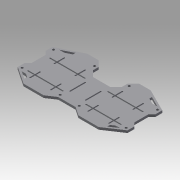
# Autodesk Inventor part: Board_Support
Saved by Autodesk Inventor 2016 (Build 200138000, 138)
## iProperties
Created: 2015-09-29
Part Number: Board_Support
Material: Générique
Document SubType Name: Modeling
Designer: Logan
Density: 1 g/cm^3
Appearance: Par défaut
Author: Logan
Autodesk Inventor part; units mm, degrees
ref_plane "YZ Plane" through (0, 0, 0) normal (1, 0, 0) x (0, 1, 0)
ref_plane "XZ Plane" through (0, 0, 0) normal (0, 1, 0) x (-1, 0, 0)
ref_plane "XY Plane" through (0, 0, 0) normal (0, 0, 1) x (1, 0, 0)
sketch "Esquisse1" plane through (0, 0, 0) normal (0, 0, 1) x (1, 0, 0)
  line L0 (-190, -60) -> (-190, 60)
  line L1 (190, 60) -> (190, -60)
  line L2 (-110, 100) -> (-190, 60)
  line L3 (110, 100) -> (190, 60)
  line L4 (-190, -60) -> (-130, -100)
  line L5 (130, -100) -> (190, -60)
  line L6 (70, 100) -> (110, 100)
  line L7 (130, -100) -> (60, -100)
  line L8 (-60, -100) -> (-130, -100)
  line L9 (30, 40) -> (-30, 40)
  line L10 (-110, 100) -> (-70, 100)
  line L11 (60, 100) -> (110, 100)
  line L12 (-60, -100) -> (-30, -80)
  line L13 (-30, -80) -> (30, -80)
  line L14 (30, -80) -> (60, -100)
  line L15 (-50, 60) -> (-50, 80)
  line L16 (50, 60) -> (50, 80)
  line L17 (-30, 40) -> (-50, 60)
  line L18 (30, 40) -> (50, 60)
  line L19 (-70, 100) -> (-50, 80)
  line L20 (70, 100) -> (50, 80)
  point P0 (0, 0)
  point P1 (-60, 100)
  point P2 (-50, 40)
  point P3 (50, 40)
  point P4 (-50, 100)
  point P5 (50, 100)
  dimension "d204" = 60
  dimension "d207" = 50
  dimension "d208" = 50
  dimension "d211" = 20
  dimension "d212" = 30
  dimension "d213" = 30
  dimension "d214" = 20
  dimension "d215" = 20
  dimension "d216" = 20
  dimension "d217" = 20
  dimension "d218" = 20
  dimension "d219" = 20
  dimension "d220" = 20
  dimension "d221" = 20
  dimension "d227" = 80
  dimension "d228" = 40
  dimension "d229" = 60
  dimension "d230" = 40
  dimension "d231" = 80
  dimension "d232" = 40
  dimension "d233" = 60
  dimension "d234" = 380
  dimension "d235" = 190
  dimension "d236" = 30
  dimension "d250" = 60
  dimension "d251" = 40
  constraints: 42 end point, 10 point on line, 7 parallel, 3 horizontal, 2 collinear, 2 perpendicular, 2 vertical
  measures "d204" distance between parallel lines of L9 L10
  measures "d207" horizontal distance of point (0, 0) point (50, 40)
  measures "d208" horizontal distance of point (0, 0) point (-50, 40)
  measures "d211" distance between parallel lines of L8 L13
  measures "d212" horizontal distance of L12.end L8.start
  measures "d213" horizontal distance of L7.end L13.end
  measures "d214" distance of L9.end point (-50, 40)
  measures "d215" distance of L15.start point (-50, 40)
  measures "d216" distance of L9.start point (50, 40)
  measures "d217" distance of L16.start point (50, 40)
  measures "d218" distance of L10.end point (-50, 100)
  measures "d219" distance of L15.end point (-50, 100)
  measures "d220" distance of L6.start point (50, 100)
  measures "d221" distance of L16.end point (50, 100)
  measures "d227" horizontal distance of L2.start L0.end
  measures "d228" vertical distance of L2.start L0.end
  measures "d229" horizontal distance of L0.start L4.end
  measures "d230" vertical distance of L0.start L4.end
  measures "d231" horizontal distance of L3.start L1.start
  measures "d232" vertical distance of L3.start L1.start
  measures "d233" distance of L12.end L13.end
  measures "d234" distance between parallel lines of L1 L0
  measures "d235" distance from line of point (0, 0) L0
  measures "d236" horizontal distance of point (0, 0) L13.end
  measures "d250" horizontal distance of L5.start L1.end
  measures "d251" vertical distance of L5.start L1.end
extrude "Plaque" add sketch "Esquisse1" along normal blind 8
sketch "Esquisse8" plane through (0, 0, 8) normal (0, 0, 1) x (1, 0, 0)
  line L0 (-178, -30) -> (-190, -30)
  line L1 (-190, -30) -> (-190, 30)
  line L2 (-190, 30) -> (-178, 30)
  line L3 (-178, 30) -> (-178, -30)
  line L4 (-178, -30) -> (-190, 30) construction
  line L5 (-190, -30) -> (-178, 30) construction
  line L6 (0, 43.7993) -> (0, -83.0015)
  line L7 (178, -30) -> (190, -30)
  line L8 (190, -30) -> (190, 30)
  line L9 (190, 30) -> (178, 30)
  line L10 (178, 30) -> (178, -30)
  line L11 (178, -30) -> (190, 30) construction
  line L12 (190, -30) -> (178, 30) construction
  point P0 (0, 0)
  point P1 (-184, 0)
  point P2 (184, 0)
  dimension "d106" = 60
  dimension "d107" = 12
  dimension "d108" = 178
  dimension "d191" = 30
  constraints: 26 end point, 5 symmetric about line, 4 midpoint, 2 parallel, 1 horizontal, 1 perpendicular, 1 vertical
  measures "d106" distance of L2.end L0.start
  measures "d107" distance of L1.end L2.end
  measures "d108" distance from line of point (0, 0) L3
  measures "d191" distance from line of point (0, 0) L2
extrude "Passage_Encodeur" cut sketch "Esquisse8" against normal up to surface (8 mm away)
chamfer "Passage_cable" distance 6 angle 45 8 edges at (-178, 30, 4) (-178, -30, 4) (178, 30, 4) (178, -30, 4) (190, 30, 4) (-190, 30, 4) (-190, -30, 4) (190, -30, 4)
sketch "Esquisse12" plane through (0, 0, 8) normal (0, 0, 1) x (1, 0, 0)
  line L0 (178, -24) -> (190, -36) projected
  line L1 (178, -24) -> (178, 24) projected
  line L2 (190, 36) -> (178, 24) projected
  line L3 (190, 36) -> (190, 60) projected
  line L4 (190, 60) -> (110, 100) projected
  line L5 (110, 100) -> (70, 100) projected
  line L6 (70, 100) -> (50, 80) projected
  line L7 (50, 80) -> (50, 60) projected
  line L8 (50, 60) -> (30, 40) projected
  line L9 (30, 40) -> (-30, 40) projected
  line L10 (-30, 40) -> (-50, 60) projected
  line L11 (-50, 60) -> (-50, 80) projected
  line L12 (-50, 80) -> (-70, 100) projected
  line L13 (-70, 100) -> (-110, 100) projected
  line L14 (-110, 100) -> (-190, 60) projected
  line L15 (-190, 60) -> (-190, 36) projected
  line L16 (-178, 24) -> (-190, 36) projected
  line L17 (-178, 24) -> (-178, -24) projected
  line L18 (-190, -36) -> (-178, -24) projected
  line L19 (-190, -36) -> (-190, -60) projected
  line L20 (-190, -60) -> (-130, -100) projected
  line L21 (-130, -100) -> (-60, -100) projected
  line L22 (-60, -100) -> (-30, -80) projected
  line L23 (-30, -80) -> (30, -80) projected
  line L24 (30, -80) -> (60, -100) projected
  line L25 (60, -100) -> (130, -100) projected
  line L26 (130, -100) -> (190, -60) projected
  line L27 (190, -60) -> (190, -36) projected
  line L28 (-180, 53.8197) -> (-107.6393, 90)
  line L29 (-107.6393, 90) -> (-74.1421, 90)
  line L30 (-74.1421, 90) -> (-60, 75.8579)
  line L31 (-60, 75.8579) -> (-60, 55.8579)
  line L32 (-60, 55.8579) -> (-34.1421, 30)
  line L33 (-34.1421, 30) -> (34.1421, 30)
  line L34 (34.1421, 30) -> (60, 55.8579)
  line L35 (60, 55.8579) -> (60, 75.8579)
  line L36 (60, 75.8579) -> (74.1421, 90)
  line L37 (74.1421, 90) -> (107.6393, 90)
  line L38 (107.6393, 90) -> (180, 53.8197)
  line L39 (180, 53.8197) -> (180, 40.1421)
  line L40 (180, 40.1421) -> (168, 28.1421)
  line L41 (168, 28.1421) -> (168, -28.1421)
  line L42 (168, -28.1421) -> (180, -40.1421)
  line L43 (180, -40.1421) -> (180, -54.6482)
  line L44 (180, -54.6482) -> (126.9722, -90)
  line L45 (126.9722, -90) -> (63.0278, -90)
  line L46 (63.0278, -90) -> (33.0278, -70)
  line L47 (33.0278, -70) -> (-33.0278, -70)
  line L48 (-33.0278, -70) -> (-63.0278, -90)
  line L49 (-63.0278, -90) -> (-126.9722, -90)
  line L50 (-126.9722, -90) -> (-180, -54.6482)
  line L51 (-180, -54.6482) -> (-180, -40.1421)
  line L52 (-180, -40.1421) -> (-168, -28.1421)
  line L53 (-168, -28.1421) -> (-168, 28.1421)
  line L54 (-168, 28.1421) -> (-180, 40.1421)
  line L55 (-180, 40.1421) -> (-180, 53.8197)
  point P0 (0, 0)
  dimension "d263" = 10
  constraints: 56 end point, 27 other
  measures "d263" distance between parallel lines of L14 L28
hole "Support_Etage" at (-180, 53.8197, 8) at (180, 53.8197, 8) at (180, -54.6482, 8) at (-180, -54.6482, 8) at (-60, 75.8579, 8) at (60, 75.8579, 8) at (33.0278, -70, 8) at (-33.0278, -70, 8) direction (0, 0, -1) diameter 8 end through all
sketch "Esquisse16" plane through (0, 0, 8) normal (0, 0, 1) x (1, 0, 0)
  line L0 (-110, 100) -> (-190, 60) projected
  line L1 (-169.9266, 63.3285) -> (-132.3607, 82.1115)
  line L2 (-132.3607, 82.1115) -> (-132.3607, 82.1115)
  line L3 (-132.3607, 73.1672) -> (-152.0381, 63.3285)
  line L4 (-169.9266, 63.3285) -> (-169.9266, 63.3285)
  line L5 (-132.3607, 82.1115) -> (-132.3607, 73.1672)
  line L6 (-152.0381, 63.3285) -> (-169.9266, 63.3285)
  line L7 (-50, 60) -> (-50, 80) projected
  line L8 (-70, 100) -> (-110, 100) projected
  line L9 (-190, -60) -> (-130, -100) projected
  line L10 (-169.9266, -66.1711) -> (-143.301, -83.9216)
  line L11 (-143.301, -83.9216) -> (-143.301, -83.9216)
  line L12 (-143.301, -74.3068) -> (-155.5044, -66.1711)
  line L13 (-169.9266, -66.1711) -> (-169.9266, -66.1711)
  line L14 (-155.5044, -66.1711) -> (-169.9266, -66.1711)
  line L15 (-143.301, -83.9216) -> (-143.301, -74.3068)
  line L16 (-190, -36) -> (-190, -60) projected
  line L17 (-130, -100) -> (-60, -100) projected
  line L18 (0, 0) -> (0, -41.1993)
  line L19 (110, 100) -> (190, 60)
  line L20 (169.9266, 63.3285) -> (132.3607, 82.1115)
  line L21 (132.3607, 82.1115) -> (132.3607, 82.1115)
  line L22 (132.3607, 73.1672) -> (152.0381, 63.3285)
  line L23 (169.9266, 63.3285) -> (169.9266, 63.3285)
  line L24 (132.3607, 82.1115) -> (132.3607, 73.1672)
  line L25 (152.0381, 63.3285) -> (169.9266, 63.3285)
  line L26 (50, 60) -> (50, 80)
  line L27 (70, 100) -> (110, 100)
  line L28 (190, -60) -> (130, -100)
  line L29 (169.9266, -66.1711) -> (143.301, -83.9216)
  line L30 (143.301, -83.9216) -> (143.301, -83.9216)
  line L31 (143.301, -74.3068) -> (155.5044, -66.1711)
  line L32 (169.9266, -66.1711) -> (169.9266, -66.1711)
  line L33 (155.5044, -66.1711) -> (169.9266, -66.1711)
  line L34 (143.301, -83.9216) -> (143.301, -74.3068)
  line L35 (190, -36) -> (190, -60)
  line L36 (130, -100) -> (60, -100)
  point P0 (-128.783, 74.956)
  point P1 (-166.3489, 56.1731)
  point P2 (-138.8634, -77.2652)
  point P3 (-165.489, -59.5147)
  point P4 (128.783, 74.956)
  point P5 (166.3489, 56.1731)
  point P6 (138.8634, -77.2652)
  point P7 (165.489, -59.5147)
  dimension "d310" = 8
  dimension "d311" = 6
  dimension "d312" = 42
  dimension "d313" = 28
  dimension "d316" = 8
  dimension "d319" = 8
  dimension "d320" = 8
  dimension "d323" = 32
  dimension "d324" = 6
  dimension "d326" = 8
  dimension "d327" = 8
  dimension "d329" = 0
  constraints: 62 end point, 25 symmetric about line, 16 point on line, 10 parallel, 2 perpendicular, 1 vertical
  measures "d310" distance between parallel lines of L1 L3
  measures "d311" distance between parallel lines of L0 L1
  measures "d312" distance between parallel lines of L2 L4
  measures "d313" distance from line of L0.start L2
  measures "d316" distance of L2.end point (-128.783, 74.956)
  measures "d319" distance of L4.start point (-166.349, 56.173)
  measures "d320" distance between parallel lines of L12 L10
  measures "d323" distance between parallel lines of L11 L13
  measures "d324" distance between parallel lines of L9 L10
  measures "d326" distance of L13.start point (-165.489, -59.515)
  measures "d327" distance of L11.end point (-138.863, -77.265)
  measures "d329" horizontal distance of L1.start L10.start
extrude "Extrusion6" cut sketch "Esquisse16" against normal up to next
sketch "Esquisse17" plane through (0, 0, 8) normal (0, 0, 1) x (1, 0, 0)
  line L0 (160.48, 22.48) -> (160.48, -53.72)
  line L1 (-30, -80) -> (30, -80) projected
  line L2 (30, 40) -> (-30, 40) projected
  line L3 (178, -24) -> (178, 24) projected
  line L4 (-178, 24) -> (-178, -24) projected
  line L5 (-160.48, 22.48) -> (-40.48, 22.48) construction
  line L6 (-160.48, 20.48) -> (-40.48, 20.48)
  line L7 (-40.48, 24.48) -> (-160.48, 24.48)
  arc A0 (-160.48, 24.48) -> (-160.48, 20.48) centre (-160.48, 22.48) ccw
  arc A1 (-40.48, 20.48) -> (-40.48, 24.48) centre (-40.48, 22.48) ccw
  line L8 (-160.48, -53.72) -> (-40.48, -53.72) construction
  line L9 (-160.48, -55.72) -> (-40.48, -55.72)
  line L10 (-40.48, -51.72) -> (-160.48, -51.72)
  arc A2 (-160.48, -51.72) -> (-160.48, -55.72) centre (-160.48, -53.72) ccw
  arc A3 (-40.48, -55.72) -> (-40.48, -51.72) centre (-40.48, -53.72) ccw
  line L11 (0, 0) -> (0, -19.5991)
  line L12 (-40.48, 24.48) -> (-40.48, 20.48)
  line L13 (-40.48, -51.72) -> (-40.48, -55.72)
  line L14 (-160.48, -53.72) -> (-160.48, -51.72)
  line L15 (-160.48, 20.48) -> (-160.48, 22.48)
  line L16 (-160.48, 22.48) -> (-40.48, 22.48)
  line L17 (-40.48, -53.72) -> (-160.48, -53.72)
  line L18 (160.48, 22.48) -> (40.48, 22.48) construction
  line L19 (160.48, 20.48) -> (40.48, 20.48)
  line L20 (40.48, 24.48) -> (160.48, 24.48)
  arc A4 (160.48, 20.48) -> (160.48, 24.48) centre (160.48, 22.48) ccw
  arc A5 (40.48, 24.48) -> (40.48, 20.48) centre (40.48, 22.48) ccw
  line L21 (160.48, -53.72) -> (40.48, -53.72) construction
  line L22 (160.48, -55.72) -> (40.48, -55.72)
  line L23 (40.48, -51.72) -> (160.48, -51.72)
  arc A6 (160.48, -55.72) -> (160.48, -51.72) centre (160.48, -53.72) ccw
  arc A7 (40.48, -51.72) -> (40.48, -55.72) centre (40.48, -53.72) ccw
  line L24 (40.48, 24.48) -> (40.48, 20.48)
  line L25 (40.48, -51.72) -> (40.48, -55.72)
  line L26 (160.48, -53.72) -> (160.48, -51.72)
  line L27 (160.48, 20.48) -> (160.48, 22.48)
  line L28 (160.48, 22.48) -> (40.48, 22.48)
  line L29 (40.48, -53.72) -> (160.48, -53.72)
  point P0 (-100.48, 22.48)
  point P1 (-100.48, -53.72)
  point P2 (100.48, 22.48)
  point P3 (100.48, -53.72)
  dimension "d334" = 17.52
  dimension "d337" = 4
  dimension "d338" = 4
  constraints: 60 end point, 16 point on circle, 12 symmetric about line, 8 centre point, 8 tangent, 6 midpoint, 5 parallel, 3 vertical, 1 horizontal, 1 perpendicular, 4 other
  measures "d334" distance between parallel lines of L3 L0
  measures "d337" diameter of A1
  measures "d338" diameter of A3
extrude "Extrusion7" cut sketch "Esquisse17" against normal up to next
sketch "Esquisse18" plane through (0, 0, 8) normal (0, 0, 1) x (1, 0, 0)
  line L0 (-26.9867, 10.48) -> (-26.9867, -41.72)
  line L1 (0, 0) -> (0, -20.4162)
  arc A0 (-40.48, 20.48) -> (-40.48, 24.48) centre (-40.48, 22.48) ccw projected
  line L2 (-40.48, 20.48) -> (-160.48, 20.48) projected
  line L3 (-160.48, -51.72) -> (-40.48, -51.72) projected
  line L4 (26.9867, 10.48) -> (26.9867, -41.72)
  line L5 (-26.9867, 10.48) -> (-26.9867, -41.72) construction
  line L6 (-28.9867, 10.48) -> (-28.9867, -41.72)
  line L7 (-24.9867, -41.72) -> (-24.9867, 10.48)
  arc A1 (-24.9867, 10.48) -> (-28.9867, 10.48) centre (-26.9867, 10.48) ccw
  arc A2 (-28.9867, -41.72) -> (-24.9867, -41.72) centre (-26.9867, -41.72) ccw
  line L8 (26.9867, 10.48) -> (26.9867, -41.72) construction
  line L9 (24.9867, 10.48) -> (24.9867, -41.72)
  line L10 (28.9867, -41.72) -> (28.9867, 10.48)
  arc A3 (28.9867, 10.48) -> (24.9867, 10.48) centre (26.9867, 10.48) ccw
  arc A4 (24.9867, -41.72) -> (28.9867, -41.72) centre (26.9867, -41.72) ccw
  point P0 (-26.9867, -15.62)
  point P1 (26.9867, -15.62)
  dimension "d341" = 26.9867
  dimension "d342" = 13.4933
  dimension "d343" = 10
  dimension "d344" = 10
  dimension "d345" = 4
  dimension "d346" = 4
  constraints: 22 end point, 8 point on circle, 8 tangent, 4 centre point, 3 equal length, 3 vertical, 2 midpoint, 2 symmetric about line
  measures "d341" distance between parallel lines of L1 L0
  measures "d342" distance from line of A0.centre L0
  measures "d343" distance from line of L2 L0.start
  measures "d344" distance from line of L3 L0.end
  measures "d345" diameter of A2
  measures "d346" diameter of A4
extrude "Extrusion8" cut sketch "Esquisse18" against normal up to next
sketch "Esquisse19" plane through (0, 0, 8) normal (0, 0, 1) x (1, 0, 0)
  line L0 (-136.58, 47.7) -> (-64.38, 47.7)
  line L1 (-64.38, 47.7) -> (-64.38, 13.26)
  line L2 (-64.38, 13.26) -> (-136.58, 13.26)
  line L3 (-136.58, 13.26) -> (-136.58, 47.7)
  line L4 (24.9867, -41.72) -> (24.9867, 10.48) projected
  line L5 (-24.9867, 10.48) -> (-24.9867, -41.72) projected
  arc A0 (-40.48, 20.48) -> (-40.48, 24.48) centre (-40.48, 22.48) ccw projected
  arc A1 (-160.48, 24.48) -> (-160.48, 20.48) centre (-160.48, 22.48) ccw projected
  line L6 (-160.48, -51.72) -> (-40.48, -51.72) projected
  line L7 (-40.48, 20.48) -> (-160.48, 20.48) projected
  line L8 (-160.48, 24.48) -> (-40.48, 24.48) projected
  line L9 (0, 0) -> (0, -36.2829)
  line L10 (136.58, 47.7) -> (64.38, 47.7)
  line L11 (64.38, 47.7) -> (64.38, 13.26)
  line L12 (64.38, 13.26) -> (136.58, 13.26)
  line L13 (136.58, 13.26) -> (136.58, 47.7)
  line L14 (-136.58, 47.7) -> (-136.58, 13.26) construction
  line L15 (-138.58, 47.7) -> (-138.58, 13.26)
  line L16 (-134.58, 13.26) -> (-134.58, 47.7)
  arc A2 (-134.58, 47.7) -> (-138.58, 47.7) centre (-136.58, 47.7) ccw
  arc A3 (-138.58, 13.26) -> (-134.58, 13.26) centre (-136.58, 13.26) ccw
  line L17 (-64.38, 47.7) -> (-64.38, 13.26) construction
  line L18 (-66.38, 47.7) -> (-66.38, 13.26)
  line L19 (-62.38, 13.26) -> (-62.38, 47.7)
  arc A4 (-62.38, 47.7) -> (-66.38, 47.7) centre (-64.38, 47.7) ccw
  arc A5 (-66.38, 13.26) -> (-62.38, 13.26) centre (-64.38, 13.26) ccw
  line L20 (64.38, 47.7) -> (64.38, 13.26) construction
  line L21 (62.38, 47.7) -> (62.38, 13.26)
  line L22 (66.38, 13.26) -> (66.38, 47.7)
  arc A6 (66.38, 47.7) -> (62.38, 47.7) centre (64.38, 47.7) ccw
  arc A7 (62.38, 13.26) -> (66.38, 13.26) centre (64.38, 13.26) ccw
  line L23 (136.58, 13.26) -> (136.58, 47.7) construction
  line L24 (138.58, 13.26) -> (138.58, 47.7)
  line L25 (134.58, 47.7) -> (134.58, 13.26)
  arc A8 (134.58, 13.26) -> (138.58, 13.26) centre (136.58, 13.26) ccw
  arc A9 (138.58, 47.7) -> (134.58, 47.7) centre (136.58, 47.7) ccw
  line L26 (-7.6752, -11.52) -> (17.069, -11.52)
  line L27 (-136.58, -70.74) -> (-64.38, -70.74)
  line L28 (-64.38, -70.74) -> (-64.38, -36.3)
  line L29 (-64.38, -36.3) -> (-136.58, -36.3)
  line L30 (-136.58, -36.3) -> (-136.58, -70.74)
  line L31 (64.38, -70.74) -> (64.38, -36.3)
  line L32 (136.58, -70.74) -> (64.38, -70.74)
  line L33 (136.58, -36.3) -> (136.58, -70.74)
  line L34 (64.38, -36.3) -> (136.58, -36.3)
  line L35 (-136.58, -70.74) -> (-136.58, -36.3) construction
  line L36 (-138.58, -70.74) -> (-138.58, -36.3)
  line L37 (-134.58, -36.3) -> (-134.58, -70.74)
  arc A10 (-138.58, -70.74) -> (-134.58, -70.74) centre (-136.58, -70.74) ccw
  arc A11 (-134.58, -36.3) -> (-138.58, -36.3) centre (-136.58, -36.3) ccw
  line L38 (-64.38, -70.74) -> (-64.38, -36.3) construction
  line L39 (-66.38, -70.74) -> (-66.38, -36.3)
  line L40 (-62.38, -36.3) -> (-62.38, -70.74)
  arc A12 (-66.38, -70.74) -> (-62.38, -70.74) centre (-64.38, -70.74) ccw
  arc A13 (-62.38, -36.3) -> (-66.38, -36.3) centre (-64.38, -36.3) ccw
  line L41 (64.38, -70.74) -> (64.38, -36.3) construction
  line L42 (62.38, -70.74) -> (62.38, -36.3)
  line L43 (66.38, -36.3) -> (66.38, -70.74)
  arc A14 (62.38, -70.74) -> (66.38, -70.74) centre (64.38, -70.74) ccw
  arc A15 (66.38, -36.3) -> (62.38, -36.3) centre (64.38, -36.3) ccw
  line L44 (136.58, -36.3) -> (136.58, -70.74) construction
  line L45 (138.58, -36.3) -> (138.58, -70.74)
  line L46 (134.58, -70.74) -> (134.58, -36.3)
  arc A16 (138.58, -36.3) -> (134.58, -36.3) centre (136.58, -36.3) ccw
  arc A17 (134.58, -70.74) -> (138.58, -70.74) centre (136.58, -70.74) ccw
  point P0 (-136.58, 30.48)
  point P1 (-64.38, 30.48)
  point P2 (64.38, 30.48)
  point P3 (136.58, 30.48)
  point P4 (-136.58, -53.52)
  point P5 (-64.38, -53.52)
  point P6 (64.38, -53.52)
  point P7 (136.58, -53.52)
  dimension "d251" = 40
  dimension "d351" = 23.9
  dimension "d352" = 23.9
  dimension "d353" = 72.2
  dimension "d354" = 64.98
  dimension "d355" = 23.22
  dimension "d356" = 4
  dimension "d357" = 4
  dimension "d358" = 4
  dimension "d359" = 4
  dimension "d370" = 72.2
  dimension "d372" = 32
  dimension "d373" = 118.44
  constraints: 100 end point, 32 point on circle, 32 symmetric about line, 16 centre point, 16 tangent, 8 equal length, 4 midpoint, 3 perpendicular, 2 horizontal, 1 vertical, 8 other
  measures "d351" distance from line of A0.centre L1
  measures "d352" distance from line of A1.centre L3
  measures "d353" distance between parallel lines of L6 L7
  measures "d354" distance between parallel lines of L6 L2
  measures "d355" distance between parallel lines of L8 L0
  measures "d356" diameter of A3
  measures "d357" diameter of A5
  measures "d358" diameter of A7
  measures "d359" diameter of A9
  measures "d370" distance between parallel lines of L1 L3
  measures "d372" distance between parallel lines of L26 L7
  measures "d373" distance between parallel lines of L27 L0
extrude "Extrusion9" cut sketch "Esquisse19" against normal up to next contours L3 L8 L15 A2 L0 | L0 L16 L8 L3 | L8 L16 L7 L3 | L3 L7 L15 L8 | A4 L19 L8 L1 L0 | L0 L1 L8 L18 | L7 L16 L2 L3 | L3 L2 A3 L15 L7 | L8 L1 L7 L18 | L8 L19 L7 L1 | L7 L1 L2 L18 | L7 L19 A5 L2 L1 | L36 A11 L29 L30 L6 | L6 L30 L27 A10 L36 | L30 L29 L37 L6 | L6 L37 L27 L30 | L39 L29 L28 L6 | L6 L28 L27 L39 | L27 L28 L6 L40 A12 | A13 L40 L6 L28 L29 | L13 L12 L25 L10 | L10 A9 L24 A8 L12 L13 | L22 L12 L11 L10 | L10 L11 L12 A7 L21 A6 | L32 A14 L42 A15 L34 L31 | L31 L34 L43 L32 | L46 L34 L33 L32 | L32 L33 L34 A16 L45 A17
